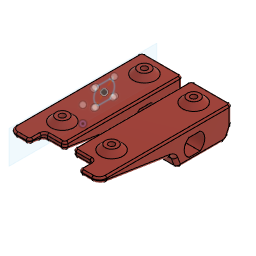
Motor mount (Autodesk Fusion 360 design; units mm, degrees)
Autodesk Fusion 360 part; units mm, degrees
sketch "Sketch1" plane through (0, 0, 0) normal (0, 0, 1) x (1, 0, 0)
  line L0 (-12.5, 45) -> (12.5, 45)
  line L1 (12.5, 45) -> (12.5, -45)
  line L2 (12.5, -45) -> (-12.5, -45)
  line L3 (-12.5, -45) -> (-12.5, 45)
  line L4 (-12.5, 45) -> (12.5, -45) construction
  line L5 (12.5, 45) -> (-12.5, -45) construction
  line L6 (0, 0) -> (0, 25) construction
  line L7 (0, 0) -> (0, -25) construction
  circle A0 centre (0, 25) radius 1.8
  circle A1 centre (0, -25) radius 1.8
  circle A2 centre (0, 25) radius 3.8
  circle A3 centre (0, -25) radius 3.8
  dimension "d1" = 25
  dimension "d2" = 90
  dimension "d3" = 25
  dimension "d4" = 25
  dimension "d5" = 3.6
  dimension "d6" = 3.6
  dimension "d28" = 2
  dimension "d29" = 2
  constraint horizontal L0
  constraint perpendicular L0 L1
  constraint parallel L0 L2
  constraint parallel L1 L3
  constraint coincident L4 L6.start
  constraint coincident L5 L6.start
  constraint coincident L6.start L7.start
  constraint parallel L3 L6
  constraint parallel L1 L7
  constraint coincident L6.end A0.centre
  constraint coincident L7.end A1.centre
  measures "d1" distance of L1.end L2.end
  measures "d2" distance of L0.end L1.end
  measures "d3" distance of L6.start L6.end
  measures "d4" distance of L6.start L7.end
  measures "d5" diameter of A0
  measures "d6" diameter of A1
extrude "Extrude1" add sketch "Sketch1" along normal blind 20 contours L0 L1 L2 L3 | A2 | A3 makes body 1
sketch "Sketch2" plane through (-12.5, 0, 0) normal (-1, 0, 0) x (0, -1, 0)
  line L0 (-45, 0) -> (45, 0)
  line L1 (45, 0) -> (45, 20)
  line L2 (45, 20) -> (-45, 20)
  line L3 (-45, 20) -> (-45, 0)
  line L4 (-19.1147, 15.2885) -> (-6.8783, 4.9885) construction
  line L5 (-6.6726, 15.2885) -> (-19.3204, 4.9885) construction
  line L6 (-9.6054, 15.3885) -> (-16.3877, 15.3885)
  line L7 (-16.3877, 4.8885) -> (-9.6054, 4.8885)
  line L8 (-7.7465, 15.3885) -> (-18.2465, 4.8885) construction
  line L9 (-18.2465, 15.3885) -> (-7.7465, 4.8885) construction
  line L10 (-18.2465, 15.3885) -> (-18.2465, 13.5297)
  line L11 (-18.2465, 6.7474) -> (-18.2465, 5.8631)
  line L12 (-7.7465, 13.5297) -> (-7.7465, 14.414)
  arc A0 (-16.3877, 15.3885) -> (-16.3877, 4.8885) centre (-12.9965, 10.1385) ccw
  arc A1 (-9.6054, 4.8885) -> (-9.6054, 15.3885) centre (-12.9965, 10.1385) ccw
  point P0 (0, 10)
  point P1 (-12.9965, 10.1385)
  point P2 (-12.9965, 10.1385)
  dimension "d13" = 10
  dimension "d14" = 12.5
  dimension "d70" = 10.5
  dimension "d71" = 10.5
  constraint coincident L4 P2
  constraint coincident L5 P2
  constraint coincident P2 P1
  constraint horizontal L6
  constraint perpendicular L6 L10
  constraint parallel L6 L7
  constraint coincident L8 P2
  constraint coincident L9 P2
  constraint coincident L10.end A0
  constraint coincident L11.start A0
  constraint collinear L10 L11
  constraint coincident L12.start A0
  constraint coincident L5 L12.end
  constraint concentric A0 A1
  constraint coincident L5 L11.end
  measures "d13" distance of origin P0
  measures "d14" diameter of A0
  measures "d70" distance of L8.end L9.end
  measures "d71" distance of L9.start L8.end
extrude "Extrude3" cut sketch "Sketch2" against normal blind 31 contours L6 L7 A0 A1 bodies 1
sketch "Sketch3" plane through (-12.5, 0, 0) normal (-1, 0, 0) x (0, -1, 0)
  line L0 (45, 17) -> (0, 10)
  line L1 (0, 10) -> (-3, 2)
  line L2 (-3, 2) -> (-13, 2)
  line L3 (-13, 2) -> (-33, 2)
  line L4 (-33, 2) -> (-36, 9)
  line L5 (-36, 9) -> (-36, 20)
  line L6 (-36, 20) -> (45, 20)
  line L7 (45, 20) -> (45, 17)
  line L8 (-36, 20) -> (-45, 20)
  line L9 (-45, 20) -> (-45, 0)
  line L10 (-45, 0) -> (45, 0)
  line L11 (45, 0) -> (45, 17)
  constraint vertical L5
  constraint perpendicular L5 L6
  constraint parallel L5 L7
  constraint perpendicular L5 L8
  constraint perpendicular L6 L9
  constraint perpendicular L9 L10
  constraint perpendicular L10 L11
extrude "Extrude4" cut sketch "Sketch3" against normal blind 31 contours L0 L1 L2 L3 L4 L5 L8 L9 L10 L11 bodies 1
fillet "Fillet1" radius 4 1 edges at (0, 0, 10) on bodies 1
fillet "Fillet2" radius 4 1 edges at (0, 33, 2) on bodies 1
fillet "Fillet3" radius 4 1 edges at (0, 36, 9) on bodies 1
sketch "Sketch4" plane through (0, 0, 20) normal (0, 0, 1) x (-1, 0, 0)
  circle A0 centre (0, -25) radius 1.8
  circle A1 centre (0, 25) radius 1.8
  line L0 (-12.5, -36) -> (12.5, -36)
  line L1 (12.5, -36) -> (12.5, 45)
  line L2 (12.5, 45) -> (-12.5, 45)
  line L3 (-12.5, 45) -> (-12.5, -36)
  circle A2 centre (0, -25) radius 3.8
  circle A3 centre (0, 25) radius 3.8
  dimension "d30" = 2
  dimension "d31" = 2
extrude "Extrude5" add sketch "Sketch4" along normal blind 3 contours A2 | A3 bodies 1
chamfer "Chamfer1" distance 3 angle 45 2 edges at (3.5428, 23.6259, 20) (3.5428, -26.3741, 20) on bodies 1
sketch "Sketch5" plane through (12.5, 0, 0) normal (1, 0, 0) x (0, 1, 0)
  line L0 (36, 20) -> (-45, 20)
  arc A0 (16.3877, 4.8885) -> (16.3877, 15.3885) centre (12.9965, 10.1385) ccw
  line L1 (-32.0733, 16.0012) -> (-18, 16.0012)
  line L2 (-18, 16.0012) -> (-18, 12)
  line L3 (-18, 12) -> (-32.0733, 12)
  line L4 (-32.0733, 12) -> (-32.0733, 16.0012)
  arc A1 (35.6766, 8.2454) -> (36, 9.821) centre (32, 9.821) ccw
  line L5 (36, 9.821) -> (36, 20)
  line L6 (-45, 20) -> (-45, 17)
  line L7 (-45, 17) -> (-2.3097, 10.3593)
  arc A2 (0.8208, 7.8113) -> (-2.3097, 10.3593) centre (-2.9246, 6.4068) ccw
  line L8 (0.8208, 7.8113) -> (3, 2)
  line L9 (3, 2) -> (30.3624, 2)
  arc A3 (30.3624, 2) -> (34.039, 4.4243) centre (30.3624, 6) ccw
  line L10 (34.039, 4.4243) -> (35.6766, 8.2454)
  line L11 (9.6054, 15.3885) -> (16.3877, 15.3885)
  line L12 (16.3877, 4.8885) -> (9.6054, 4.8885)
  arc A4 (9.6054, 15.3885) -> (9.6054, 4.8885) centre (12.9965, 10.1385) ccw
  constraint horizontal L1
  constraint vertical L2
  constraint horizontal L3
  constraint vertical L4
extrude "Extrude6" cut sketch "Sketch5" along normal blind -19 and the other way blind 6 contours L2 L3 L4 L7 | L1 L2 L4 L7 bodies 1
fillet "Fillet5" radius 1 3 edges at (0, -18, 12.8) (6.5, -25.0367, 13.8946) (-6.5, -25.0367, 13.8946) on bodies 1
fillet "Fillet5" radius 1 1 edges at (0, -32.0733, 14.9892) on bodies 1
fillet "Fillet6" radius 4.5 1 edges at (-12.5, -45, 18.5) on bodies 1
sketch "Sketch6" plane through (0, 0, 20) normal (0, 0, 1) x (-1, 0, 0)
  circle A0 centre (0, 25) radius 6.8
  arc A1 (12.5, 40.5) -> (8, 45) centre (8, 40.5) ccw
  line L0 (8, 45) -> (-12.5, 45)
  line L1 (-12.5, 45) -> (-12.5, -36)
  line L2 (-12.5, -36) -> (12.5, -36)
  line L3 (12.5, -36) -> (12.5, 40.5)
  circle A2 centre (0, -25) radius 6.8
  line L4 (-12.5, 45) -> (0, 45)
  line L5 (0, 45) -> (0, 36)
  line L6 (0, 36) -> (-12.5, 36)
  line L7 (-12.5, 36) -> (-12.5, 45)
  constraint horizontal L4
  constraint vertical L5
  constraint horizontal L6
  constraint vertical L7
  constraint coincident L0.end L1.start
extrude "Extrude7" cut sketch "Sketch6" against normal blind 8 contours L0 L1 L4 L5 L6 L7 bodies 1
fillet "Fillet7" radius 2 1 edges at (0, -45, 18.5) on bodies 1
fillet "Fillet8" radius 2 1 edges at (0, -36, 17.8) on bodies 1
fillet "Fillet9" radius 2 1 edges at (12.5, -36, 17.8) on bodies 1
fillet "Fillet10" radius 2 13 edges at (-12.5, 1.9104, 4.9057) (-12.5, -0.3995, 9.5091) (-12.5, -21.4049, 13.3296) (-11.182, -43.682, 16.795) (-5, -45, 17) (-0.5858, -44.4142, 16.9089) (0, -40.5, 16.3) (0.5858, -36.5858, 15.6911) (6.25, -36, 15.6) (11.9142, -35.4142, 15.5089) (12.5, -18.1549, 12.8241) (12.5, -0.3995, 9.5091) (12.5, 1.9104, 4.9057) on bodies 1
fillet "Fillet11" radius 2 13 edges at (-12.5, 36, 14.9105) (-12.5, 35.9183, 9.0168) (-12.5, 34.8578, 6.3348) (-12.5, 32.5644, 2.6606) (-12.5, 17.7492, 2) (-11.9142, 3.6256, 2) (0, 3, 2) (11.9142, 3.6256, 2) (12.5, 17.7492, 2) (12.5, 32.5644, 2.6606) (12.5, 34.8578, 6.3348) (12.5, 35.9183, 9.0168) (12.5, 36, 14.9105) on bodies 1
fillet "Fillet12" radius 1 12 edges at (-11.182, -43.682, 20) (-5, -45, 20) (-0.5858, -44.4142, 20) (0, -40.5, 20) (0.5858, -36.5858, 20) (6.25, -36, 20) (11.9142, -35.4142, 20) (12.5, 0, 20) (11.9142, 35.4142, 20) (0, 36, 20) (-11.9142, 35.4142, 20) (-12.5, -3.25, 20) on bodies 1
ref_plane "WorkPlane1" through (26, 0, 0) normal (1, 0, 0) x (0, 1, 0)
mirror "Mirror1" about plane through (26, 0, 0) normal (1, 0, 0) of bodies 1 makes body 2
move_body "Move1" bodies 2 to x (1, 0, 0) y (0, 1, 0) z (0, 0, 1) at (-17, 0, 0)
move_body "Move2" bodies 2 to x (1, 0, 0) y (0, 1, 0) z (0, 0, 1) at (-5, 0, 0)
sketch "Sketch7" plane through (0, 36, 0) normal (0, 1, 0) x (-1, 0, 0)
  line L0 (-19.5, 19) -> (-40.5, 19)
  line L1 (-40.5, 19) -> (-40.5, 9.821)
  line L2 (-40.5, 9.821) -> (-19.5, 9.821)
  line L3 (-19.5, 9.821) -> (-19.5, 19)
  line L4 (-40, 11) -> (-20, 11) construction
  line L5 (-20, 11) -> (-20, 18) construction
  line L6 (-20, 18) -> (-40, 18) construction
  line L7 (-40, 18) -> (-40, 11) construction
  dimension "d62" = 3
  text T0 "How's My" font "Arial" height 3 align centre middle in box 20 x 7 at (-40, 11) x (1, 0) y (0, 1) spacing 1 kerned
sketch "Sketch8" plane through (0, 36, 0) normal (0, 1, 0) x (-1, 0, 0)
  line L0 (10.5, 19) -> (-10.5, 19)
  line L1 (-10.5, 19) -> (-10.5, 9.821)
  line L2 (-10.5, 9.821) -> (10.5, 9.821)
  line L3 (10.5, 9.821) -> (10.5, 19)
  line L4 (-9.5058, 11) -> (9, 11) construction
  line L5 (9, 11) -> (9, 18.0375) construction
  line L6 (9, 18.0375) -> (-9.5058, 18.0375) construction
  line L7 (-9.5058, 18.0375) -> (-9.5058, 11) construction
  dimension "d63" = 3
  text T0 "Driving?" font "Arial" height 3 align centre middle in box 18.5058 x 7.0375 at (-9.5058, 11) x (1, 0) y (0, 1) spacing 1 kerned
extrude "Extrude8" cut sketch "Sketch8" against normal blind 1 text T0 bodies 1
extrude "Extrude9" cut sketch "Sketch7" against normal blind 1 text T0 bodies 2
